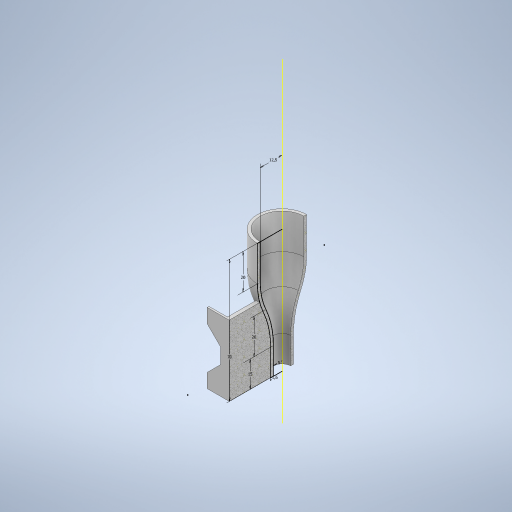
# Autodesk Inventor part: rurka_optv2
Saved by Autodesk Inventor 2023 (Build 270158000, 158)
## iProperties
Created: 2023-04-12
Part Number: rurka_optv2
Material: Ogólny
Document SubType Name: Modeling
Designer: kamil
Density: 1 g/cm^3
Appearance: Domyślna
Author: kamil
Autodesk Inventor part; units mm, degrees
ref_plane "YZ Plane" through (0, 0, 0) normal (1, 0, 0) x (0, 1, 0)
ref_plane "XZ Plane" through (0, 0, 0) normal (0, 1, 0) x (-1, 0, 0)
ref_plane "XY Plane" through (0, 0, 0) normal (0, 0, 1) x (1, 0, 0)
sketch "Szkic1" plane through (0, 0, 0) normal (1, 0, 0) x (0, 1, 0)
  line L0 (70, 12.5) -> (50, 12.5)
  arc A0 (50, 12.5) -> (35, 9.2857) centre (50, -24.1071) ccw
  arc A1 (15, 5) -> (35, 9.2857) centre (15, 53.8095) ccw
  line L1 (15, 5) -> (0, 5)
  line L2 (0.9785, 0) -> (128.1793, 0) construction
  line L3 (70, 14.1) -> (50, 14.1)
  arc A2 (50, 14.1) -> (34.3444, 10.7452) centre (50, -24.1071) ccw
  arc A3 (15, 6.6) -> (34.3444, 10.7452) centre (15, 53.8095) ccw
  line L4 (15, 6.6) -> (0, 6.6)
  line L5 (70, 14.1) -> (70, 12.5)
  line L6 (0, 6.6) -> (0, 5)
  line L7 (-25.6359, 0) -> (153.8152, 0) projected
  line L8 (70, 14.1) -> (70, 0)
  line L9 (0, 0) -> (0, 5)
  dimension "d35" = 5
  dimension "d36" = 12.5
  dimension "d37" = 70
  dimension "d38" = 20
  dimension "d39" = 15
  dimension "d40" = 20
  dimension "d41" = 1.6
  constraints: 18 end point, 8 point on circle, 4 centre point, 3 horizontal, 3 tangent, 2 parallel, 1 horizontal alignment, 1 perpendicular, 1 point on line, 1 vertical, 1 vertical alignment, 3 other
  measures "d35" distance between parallel lines of L2 L1
  measures "d36" distance between parallel lines of L2 L0
  measures "d37" horizontal distance of L1.end L0.start
  measures "d38" distance of L0.start L0.end
  measures "d39" distance of L1.start L1.end
  measures "d40" horizontal distance of L1.start A0.end
  measures "d41" distance of L4.end L1.end
revolve "Obrót1" add sketch "Szkic1" angle 360 about axis through (0, -10, 0) along (0, 1, 0) contours L0 A0 A1 L1 L6 L4 A3 A2 L3 L5
sketch "Szkic3" plane through (0, 0, 0) normal (0, 1, 0) x (-1, 0, 0)
  line L0 (2.1408, 6.3327) -> (-1.8592, 6.3327)
  line L1 (-1.8592, 6.3327) -> (-1.8592, 28.95)
  line L2 (-1.8592, 28.95) -> (2.1408, 28.95)
  line L3 (2.1408, 28.95) -> (2.1408, 6.3327)
  line L4 (-12.3592, 30) -> (12.6408, 30)
  line L5 (12.6408, 30) -> (12.6408, 28.95)
  line L6 (12.6408, 28.95) -> (-12.3592, 28.95)
  line L7 (-12.3592, 28.95) -> (-12.3592, 30)
  circle A0 centre (0, 0) radius 12.5 projected
  line L8 (2.1408, 12.3153) -> (-1.8592, 12.361)
  circle A1 centre (0, 0) radius 6.6 projected
  point P0 (0.1408, 28.95)
  point P1 (0.1408, 30)
  point P2 (2.1408, 28.95)
  point P3 (-1.8592, 28.95)
  dimension "d17" = 4
  dimension "d19" = 1.05
  dimension "d20" = 25
  dimension "d21" = 30
  constraints: 18 end point, 4 parallel, 2 horizontal, 2 midpoint, 2 perpendicular, 2 point on circle, 2 point on line, 1 horizontal alignment, 1 vertical alignment, 2 other
  measures "d17" distance between parallel lines of L1 L3
  measures "d19" distance of L6.end L4.start
  measures "d20" distance of L4.start L4.end
  measures "d21" distance from line of L4 point (0, 0)
extrude "Wyciągnięcie proste2" add sketch "Szkic3" along normal blind 40 contours L2 L6 L7 L4 L5
extrude "Wyciągnięcie proste3" add sketch "Szkic3" along normal blind 40 contours L0 A1 L1 L8 L3 | L0 A1 | A0 L1 L2 L3 | L8 A0 picked at (0.2091, 6.4118)
sketch "Szkic4" plane through (0, 40, 0) normal (0, 1, 0) x (1, 0, 0)
  line L0 (-12.6408, -30) -> (12.3592, -30) projected
  line L1 (1.9943, -30) -> (-2.1408, -30)
  line L2 (-2.1408, -5) -> (1.8592, -5)
  line L3 (-2.1408, -30) -> (1.8592, -30)
  line L4 (1.8592, -30) -> (1.8592, -5)
  line L5 (1.8592, -5) -> (-2.1408, -5)
  line L6 (-2.1408, -5) -> (-2.1408, -30)
  point P0 (0, 0)
  point P1 (-2, -5)
  point P2 (-2, -5)
  point P3 (-0.1408, -30)
  dimension "d42" = 4
  dimension "d43" = 25
  constraints: 12 end point, 3 parallel, 2 horizontal, 2 midpoint, 1 perpendicular, 1 point on line
  measures "d42" distance between parallel lines of L4 L6
  measures "d43" distance of L3.end L2.end
extrude "Wyciągnięcie proste4" add sketch "Szkic4" against normal blind 1.2
sketch "Szkic5" plane through (-12.6408, 0, 30) normal (0, 0, 1) x (1, 0, 0)
  line L0 (0, 0) -> (25, 0) projected
  line L1 (0, 0) -> (0, 8)
  line L2 (0, 0) -> (0, 40) projected
  line L3 (0, 8) -> (7.5, 15.5)
  line L4 (7.5, 15.5) -> (7.5, 24.5)
  line L5 (9.5, 70) -> (9.5, 0) projected
  line L6 (7.5, 24.5) -> (0, 32)
  line L7 (0, 40) -> (25, 40) projected
  line L8 (0, 32) -> (0, 40)
  line L9 (0, 40) -> (25, 40)
  line L10 (25, 0) -> (25, 40) projected
  line L11 (25, 40) -> (25, 32)
  line L12 (25, 32) -> (17.5, 24.5)
  line L13 (17.5, 24.5) -> (17.5, 15.5)
  line L14 (17.5, 15.5) -> (25, 8)
  line L15 (25, 8) -> (25, 0)
  line L16 (0, 0) -> (25, 0)
  line L17 (12.5, 0) -> (12.5, 40) construction
  line L18 (14.4324, 40) -> (10.5676, 40) construction
  point P0 (12.6408, 0)
  dimension "d29" = 45
  dimension "d30" = 10
  dimension "d31" = 8
  dimension "d32" = 8
  constraints: 26 end point, 4 parallel, 4 point on line, 3 perpendicular, 1 midpoint, 3 other
  measures "d29" angle of L10 L14
  measures "d30" distance between parallel lines of L13 L4
  measures "d31" distance of L6.end L2.end
  measures "d32" distance of L14.end L0.end
extrude "Wyciągnięcie proste5" cut sketch "Szkic5" against normal blind 1.2 contours L2 L6 L4 L3 | L14 L13 L12 L10
revolve "Obrót2" cut sketch "Szkic1" angle 360 about axis through (0, 0.9785, 0) along (0, 1, 0) contours L8 L7 L9 L1 A1 A0 L0
